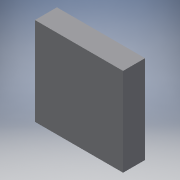
# Autodesk Inventor part: PlaceholderPart
Saved by Autodesk Inventor 2019 (Build 230136000, 136)
## iProperties
Created: 2021-09-20
Part Number: PlaceholderPart
Material: Generic
Document SubType Name: Modeling
Designer: 22spencen
Density: 1 g/cm^3
Appearance: Default
Author: 22spencen
Autodesk Inventor part; units mm, degrees
ref_plane "YZ Plane" through (0, 0, 0) normal (1, 0, 0) x (0, 1, 0)
ref_plane "XZ Plane" through (0, 0, 0) normal (0, 1, 0) x (-1, 0, 0)
ref_plane "XY Plane" through (0, 0, 0) normal (0, 0, 1) x (1, 0, 0)
sketch "Sketch1" plane through (0, 0, 0) normal (0, 0, 1) x (1, 0, 0)
  line L0 (6.35, 6.35) -> (-6.35, 6.35)
  line L1 (-6.35, 6.35) -> (-6.35, -6.35)
  line L2 (-6.35, -6.35) -> (6.35, -6.35)
  line L3 (6.35, -6.35) -> (6.35, 6.35)
  line L4 (6.35, 6.35) -> (-6.35, -6.35) construction
  line L5 (-6.35, 6.35) -> (6.35, -6.35) construction
  point P0 (0, 0)
  dimension "d0" = 12.7
  dimension "d1" = 12.7
  constraints: 12 end point, 2 midpoint, 2 parallel, 1 horizontal, 1 perpendicular
  measures "d0" distance of L2.end L1.end
  measures "d1" distance of L0.end L1.end
extrude "Extrusion1" add sketch "Sketch1" along normal blind 3.175
body "Solid1"
